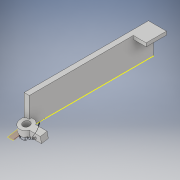
# Autodesk Inventor part: WheelIntakeMotorMount
Saved by Autodesk Inventor 2017 (Build 210142000, 142)
## iProperties
Created: 2017-11-15
Part Number: WheelIntakeMotorMount
Material: Generic
Document SubType Name: Modeling
Designer: User
Density: 1 g/cm^3
Appearance: Default
Author: User
Autodesk Inventor part; units mm, degrees
ref_plane "YZ Plane" through (0, 0, 0) normal (1, 0, 0) x (0, 1, 0)
ref_plane "XZ Plane" through (0, 0, 0) normal (0, 1, 0) x (-1, 0, 0)
ref_plane "XY Plane" through (0, 0, 0) normal (0, 0, 1) x (1, 0, 0)
sketch "Sketch2" plane through (0, 0, 0) normal (1, 0, 0) x (0, 1, 0)
  line L0 (0, 0) -> (25.4, 0)
  line L1 (25.4, 0) -> (25.4, -114.3)
  line L2 (25.4, -114.3) -> (0, -114.3)
  line L3 (0, -114.3) -> (0, 0)
  dimension "d6" = 25.4
  dimension "d7" = 114.3
  constraints: 8 end point, 2 parallel, 1 horizontal, 1 perpendicular
  measures "d6" distance of L1.end L2.end
  measures "d7" distance of L0.end L1.end
extrude "Extrusion2" add sketch "Sketch2" along normal blind 4.7625
sketch "Sketch3" plane through (4.7625, 0, 0) normal (1, 0, 0) x (0, 0, -1)
  line L0 (0, 0) -> (114.3, 0) projected
  line L1 (0, 0) -> (-14.429, -2.5442)
  line L2 (0, 0) -> (14.6516, 0) construction
  dimension "d10" = 170
  constraints: 4 end point, 1 equal length, 1 horizontal
  measures "d10" angle of L1 L2
ref_plane "Work Plane1" through (4.7625, -2.5442, 14.429) normal (0, 0.9848, 0.1736) x (0, 0.1736, -0.9848)
sketch "Sketch4" plane through (4.7625, -2.5442, 14.429) normal (0, 0.9848, 0.1736) x (0, 0.1736, -0.9848)
  line L0 (127.2151, 4.7625) -> (14.6516, 4.7625) projected
  line L1 (127.2151, 4.7625) -> (127.2151, 0) projected
  line L2 (14.6516, 0) -> (127.2151, 0) projected
  line L3 (14.6516, 4.7625) -> (14.6516, 0) projected
  arc A0 (11.4766, 4.7625) -> (14.6516, 3.9118) centre (11.4766, -1.5875) ccw
  circle A1 centre (11.4766, -1.5875) radius 3.175
  line L4 (14.6516, 4.7625) -> (11.4766, 4.7625)
  line L5 (14.6516, 4.7625) -> (14.6516, 0)
  dimension "d11" = 12.7
  dimension "d12" = 3.175
  dimension "d13" = 4.7625
  dimension "d15" = 6.35
  dimension "d26" = 1.5875
  constraints: 4 end point, 2 centre point, 2 point on circle, 1 coincident, 1 collinear, 1 horizontal, 1 point on line
  measures "d11" diameter of A0
  measures "d12" distance from line of L3 A0.centre
  measures "d13" distance of L0.end L2.start
  measures "d15" diameter of A1
  measures "d26" distance from line of L2 A0.centre
extrude "Extrusion3" add sketch "Sketch4" along normal blind 6.35 contours L3 L2 A0 L4 | A0 L2 L3
sketch "Sketch5" plane through (0, 25.4, 0) normal (0, 1, 0) x (1, 0, 0)
  line L0 (0, 0) -> (0, 114.3) projected
  line L1 (0, 0) -> (4.7625, 0) projected
  line L2 (4.7625, 114.3) -> (4.7625, 0) projected
  line L3 (0, 114.3) -> (4.7625, 114.3) projected
  line L4 (0, 114.3) -> (0, 0) projected
  line L5 (0, 114.3) -> (16.5392, 114.3)
  line L6 (16.5392, 114.3) -> (16.5392, 95.6232)
  line L7 (16.5392, 95.6232) -> (0, 95.6232)
  line L8 (0, 95.6232) -> (0, 114.3)
  constraints: 8 end point, 2 parallel, 1 horizontal, 1 perpendicular
extrude "Extrusion4" add sketch "Sketch5" against normal blind 3.175 contours L0 L3 L2 L7 | L2 L5 L6 L7
sketch "Sketch6" plane through (4.7625, -2.5442, 14.429) normal (0, 0.9848, 0.1736) x (0, 0.1736, -0.9848)
  line L0 (17.6249, 0) -> (14.6516, 0) projected
  arc A0 (17.6249, 0) -> (11.4766, 4.7625) centre (11.4766, -1.5875) ccw projected
  line L1 (14.6516, 3.9118) -> (14.6516, 0) projected
  circle A1 centre (11.4766, -1.5875) radius 3.175 projected
  line L2 (127.2151, 4.7625) -> (14.6516, 4.7625) projected
  line L3 (14.6516, -4.7625) -> (8.3016, -4.7625)
  line L4 (8.3016, -4.7625) -> (8.3016, -17.4625)
  line L5 (8.3016, -17.4625) -> (14.6516, -17.4625)
  line L6 (14.6516, -17.4625) -> (14.6516, -4.7625)
  line L7 (14.6516, 4.7625) -> (11.4766, 4.7625) projected
  line L8 (14.6516, 4.7625) -> (14.6516, 3.9118) projected
  point P0 (17.3632, 4.7625)
  dimension "d22" = 6.35
  dimension "d23" = 12.7
  dimension "d27" = 0
  constraints: 8 end point, 2 parallel, 1 horizontal, 1 perpendicular
  measures "d22" distance of L5.end L4.end
  measures "d23" distance of L4.end L3.end
  measures "d27" distance edge to line of A1 L3
extrude "Extrusion5" add sketch "Sketch6" along normal blind 6.35 contours L3 L6 L5 L4
equation "\"d26\" = 0.5 * d11 - d13"
body "Solid2"
